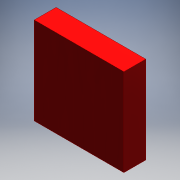
# Autodesk Inventor part: BMS
Saved by Autodesk Inventor 2016 (Build 200138000, 138)
## iProperties
Created: 2016-04-13
Part Number: BMS
Material: Generic
Document SubType Name: Modeling
Designer: agmle
Density: 1 g/cm^3
Appearance: Red
Author: agmle
Autodesk Inventor part; units mm, degrees
ref_plane "YZ Plane" through (0, 0, 0) normal (1, 0, 0) x (0, 1, 0)
ref_plane "XZ Plane" through (0, 0, 0) normal (0, 1, 0) x (-1, 0, 0)
ref_plane "XY Plane" through (0, 0, 0) normal (0, 0, 1) x (1, 0, 0)
sketch "Sketch1" plane through (0, 0, 0) normal (0, 1, 0) x (-1, 0, 0)
  line L0 (41, 40) -> (-41, 40)
  line L1 (-41, 40) -> (-41, -40)
  line L2 (-41, -40) -> (41, -40)
  line L3 (41, -40) -> (41, 40)
  line L4 (41, 0) -> (-41, 0) construction
  point P0 (0, 0)
  point P1 (0, 0)
  dimension "d0" = 80
  dimension "d1" = 82
  constraints: 10 end point, 3 midpoint, 2 parallel, 1 coincident, 1 horizontal, 1 perpendicular
  measures "d0" distance of L2.end L0.start
  measures "d1" distance of L0.start L0.end
extrude "Extrusion1" add sketch "Sketch1" along normal blind 20
body "Solid1"
